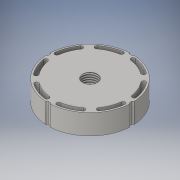
# Autodesk Inventor part: ICRC wrist model
Saved by Autodesk Inventor 2016 (Build 200138000, 138)
## iProperties
Created: 2016-04-29
Part Number: ICRC wrist model
Material: Generic
Document SubType Name: Modeling
Designer: au233088
Density: 1 g/cm^3
Appearance: Default
Author: au233088
Autodesk Inventor part; units mm, degrees
ref_plane "YZ Plane" through (0, 0, 0) normal (1, 0, 0) x (0, 1, 0)
ref_plane "XZ Plane" through (0, 0, 0) normal (0, 1, 0) x (-1, 0, 0)
ref_plane "XY Plane" through (0, 0, 0) normal (0, 0, 1) x (1, 0, 0)
sketch "Sketch1" plane through (0, 0, 0) normal (0, 1, 0) x (-1, 0, 0)
  circle A0 centre (0, 0) radius 25
  dimension "d1" = 50
  constraints: 1 centre point, 1 coincident
  measures "d1" diameter of A0
extrude "Extrusion1" add sketch "Sketch1" along normal blind 12
sketch "Sketch2" plane through (0, 12, 0) normal (0, 1, 0) x (1, 0, 0)
  circle A0 centre (0, 0) radius 1.3723
  line L0 (-24.9867, -1.3423) -> (-24.9867, 1.3423) construction
  line L1 (-24.2459, -0.6015) -> (-24.2459, 0.6015)
  line L2 (-25.7274, 0.6015) -> (-25.7274, -0.6015)
  arc A1 (-25.7274, -0.6015) -> (-24.2459, -0.6015) centre (-24.9867, -0.6015) ccw
  arc A2 (-24.2459, 0.6015) -> (-25.7274, 0.6015) centre (-24.9867, 0.6015) ccw
  line L3 (1.3423, -24.9867) -> (-1.3423, -24.9867) construction
  line L4 (0.6015, -24.2459) -> (-0.6015, -24.2459)
  line L5 (-0.6015, -25.7274) -> (0.6015, -25.7274)
  arc A3 (0.6015, -25.7274) -> (0.6015, -24.2459) centre (0.6015, -24.9867) ccw
  arc A4 (-0.6015, -24.2459) -> (-0.6015, -25.7274) centre (-0.6015, -24.9867) ccw
  line L6 (24.9867, 1.3423) -> (24.9867, -1.3423) construction
  line L7 (24.2459, 0.6015) -> (24.2459, -0.6015)
  line L8 (25.7274, -0.6015) -> (25.7274, 0.6015)
  arc A5 (25.7274, 0.6015) -> (24.2459, 0.6015) centre (24.9867, 0.6015) ccw
  arc A6 (24.2459, -0.6015) -> (25.7274, -0.6015) centre (24.9867, -0.6015) ccw
  line L9 (-1.3423, 24.9867) -> (1.3423, 24.9867) construction
  line L10 (-0.6015, 24.2459) -> (0.6015, 24.2459)
  line L11 (0.6015, 25.7274) -> (-0.6015, 25.7274)
  arc A7 (-0.6015, 25.7274) -> (-0.6015, 24.2459) centre (-0.6015, 24.9867) ccw
  arc A8 (0.6015, 24.2459) -> (0.6015, 25.7274) centre (0.6015, 24.9867) ccw
  point P0 (-24.9867, 0)
  point P1 (0, -24.9867)
  point P2 (24.9867, 0)
  point P3 (0, 24.9867)
  dimension "d11" = 360
  constraints: 32 end point, 24 point on circle, 9 centre point, 8 point on line, 4 tangent, 1 coincident, 1 midpoint, 1 parallel, 1 vertical, 57 other
extrude "Extrusion2" cut sketch "Sketch2" against normal blind 12 contours A1 L2 A2 L1 | A3 L5 A4 L4 | A5 L8 A6 L7 | A7 L11 A8 L10
sketch "Sketch3" plane through (0, 12, 0) normal (0, 1, 0) x (1, 0, 0)
  circle A0 centre (0, 0) radius 22.8086
  arc A1 (13.2024, 18.5991) -> (2.9253, 22.6202) centre (0, 0) ccw construction
  arc A2 (13.9039, 19.5873) -> (3.0807, 23.822) centre (0, 0) ccw
  arc A3 (12.501, 17.611) -> (2.7699, 21.4184) centre (0, 0) ccw
  arc A4 (12.501, 17.611) -> (13.9039, 19.5873) centre (13.2024, 18.5991) ccw
  arc A5 (3.0807, 23.822) -> (2.7699, 21.4184) centre (2.9253, 22.6202) ccw
  line L0 (0, 0) -> (13.2024, 18.5991) construction
  line L1 (0, 0) -> (2.9253, 22.6202) construction
  arc A6 (-4.0188, 23.6818) -> (-14.6663, 19.0231) centre (0, 0) ccw
  arc A7 (-14.6663, 19.0231) -> (-13.1865, 17.1037) centre (-13.9264, 18.0634) ccw
  arc A8 (-3.6133, 21.2924) -> (-13.1865, 17.1037) centre (0, 0) ccw
  arc A9 (-3.6133, 21.2924) -> (-4.0188, 23.6818) centre (-3.816, 22.4871) ccw
  arc A10 (-19.5873, 13.9039) -> (-23.822, 3.0807) centre (0, 0) ccw
  arc A11 (-23.822, 3.0807) -> (-21.4184, 2.7699) centre (-22.6202, 2.9253) ccw
  arc A12 (-17.611, 12.501) -> (-21.4184, 2.7699) centre (0, 0) ccw
  arc A13 (-17.611, 12.501) -> (-19.5873, 13.9039) centre (-18.5991, 13.2024) ccw
  arc A14 (-23.6818, -4.0188) -> (-19.0231, -14.6663) centre (0, 0) ccw
  arc A15 (-19.0231, -14.6663) -> (-17.1037, -13.1865) centre (-18.0634, -13.9264) ccw
  arc A16 (-21.2924, -3.6133) -> (-17.1037, -13.1865) centre (0, 0) ccw
  arc A17 (-21.2924, -3.6133) -> (-23.6818, -4.0188) centre (-22.4871, -3.816) ccw
  arc A18 (-13.9039, -19.5873) -> (-3.0807, -23.822) centre (0, 0) ccw
  arc A19 (-3.0807, -23.822) -> (-2.7699, -21.4184) centre (-2.9253, -22.6202) ccw
  arc A20 (-12.501, -17.611) -> (-2.7699, -21.4184) centre (0, 0) ccw
  arc A21 (-12.501, -17.611) -> (-13.9039, -19.5873) centre (-13.2024, -18.5991) ccw
  arc A22 (4.0188, -23.6818) -> (14.6663, -19.0231) centre (0, 0) ccw
  arc A23 (14.6663, -19.0231) -> (13.1865, -17.1037) centre (13.9264, -18.0634) ccw
  arc A24 (3.6133, -21.2924) -> (13.1865, -17.1037) centre (0, 0) ccw
  arc A25 (3.6133, -21.2924) -> (4.0188, -23.6818) centre (3.816, -22.4871) ccw
  arc A26 (19.5873, -13.9039) -> (23.822, -3.0807) centre (0, 0) ccw
  arc A27 (23.822, -3.0807) -> (21.4184, -2.7699) centre (22.6202, -2.9253) ccw
  arc A28 (17.611, -12.501) -> (21.4184, -2.7699) centre (0, 0) ccw
  arc A29 (17.611, -12.501) -> (19.5873, -13.9039) centre (18.5991, -13.2024) ccw
  arc A30 (23.6818, 4.0188) -> (19.0231, 14.6663) centre (0, 0) ccw
  arc A31 (19.0231, 14.6663) -> (17.1037, 13.1865) centre (18.0634, 13.9264) ccw
  arc A32 (21.2924, 3.6133) -> (17.1037, 13.1865) centre (0, 0) ccw
  arc A33 (21.2924, 3.6133) -> (23.6818, 4.0188) centre (22.4871, 3.816) ccw
  dimension "d15" = 28
  dimension "d18" = 360
  constraints: 66 point on circle, 33 centre point, 4 end point, 4 tangent, 2 coincident, 92 other
  measures "d15" angle of L0 L1
extrude "Extrusion3" cut sketch "Sketch3" against normal blind 12 contours A33 A32 A31 A0 | A0 A31 A30 A33 | A27 A26 A29 A0 | A0 A29 A28 A27 | A4 A3 A5 A0 | A0 A5 A2 A4 | A23 A22 A25 A0 | A0 A25 A24 A23 | A9 A8 A7 A0 | A0 A7 A6 A9 | A19 A18 A21 A0 | A0 A21 A20 A19 | A13 A12 A11 A0 | A0 A11 A10 A13 | A15 A14 A17 A0 | A0 A17 A16 A15
sketch "Sketch4" plane through (0, 12, 0) normal (0, 1, 0) x (1, 0, 0)
  circle A0 centre (0, 0) radius 4.43
  dimension "d22" = 8.86
  constraints: 1 centre point, 1 coincident
  measures "d22" diameter of A0
extrude "Extrusion4" cut sketch "Sketch4" against normal blind 12
thread "Thread1" size "M10x1.25" class "6H" standard "ISO Metric profile" full length
sketch "Sketch5" plane through (0, 12, 0) normal (0, 1, 0) x (1, 0, 0)
  circle A0 centre (0, 0) radius 4.43
  constraints: 1 centre point, 1 coincident
extrude "Extrusion5" [suppressed]
thread "Thread3" size "M10x1" class "6g" standard "ANSI Metric M Profile" full length
thread "Thread4" size "M10x1" class "6g" standard "ANSI Metric M Profile" full length
body "Solid1"
